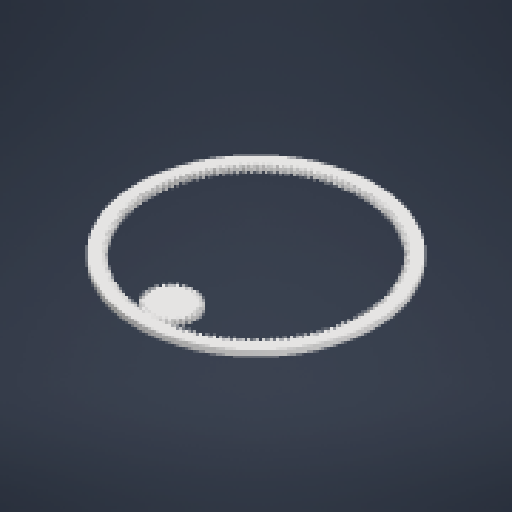
# Autodesk Inventor part: gears1
Saved by Autodesk Inventor 2026.1 (Build 301233000, 233)
## iProperties
Created: 2026-03-26
Part Number: gears1
Material: Generic
Document SubType Name: Modeling
Designer: sniel
Density: 1 g/cm^3
Appearance: Default
Author: sniel
Autodesk Inventor part; units mm, degrees
(part 1 of 2)
ref_plane "YZ Plane" through (0, 0, 0) normal (1, 0, 0) x (0, 1, 0)
ref_plane "XZ Plane" through (0, 0, 0) normal (0, 1, 0) x (-1, 0, 0)
ref_plane "XY Plane" through (0, 0, 0) normal (0, 0, 1) x (1, 0, 0)
sketch "Sketch2" plane through (0, 0, 0) normal (0, 1, 0) x (-1, 0, 0)
  arc A0 (4.4637, 88.5451) -> (4.2983, 91.7831) centre (-8.532, 89.5045) ccw
  arc A1 (4.2983, 91.7831) -> (3.1779, 92.0382) centre (-0.6449, 72.6571) ccw
  arc A2 (3.1779, 92.0382) -> (1.6272, 89.1908) centre (13.7576, 84.4303) ccw
  arc A3 (1.6272, 89.1908) -> (0.662, 89.295) centre (-0.6449, 72.6571) ccw
  arc A4 (0.662, 89.295) -> (-0.2457, 92.4075) centre (-12.2047, 87.2315) ccw
  arc A5 (-0.2457, 92.4075) -> (-1.3947, 92.3973) centre (-0.6449, 72.6571) ccw
  arc A6 (-1.3947, 92.3973) -> (-2.247, 89.2692) centre (10.6543, 87.4344) ccw
  arc A7 (-2.247, 89.2692) -> (-3.2102, 89.1479) centre (-0.6449, 72.6571) ccw
  arc A8 (-3.2102, 89.1479) -> (-4.8112, 91.9672) centre (-15.2542, 84.1728) ccw
  arc A9 (-4.8112, 91.9672) -> (-5.9269, 91.6923) centre (-0.6449, 72.6571) ccw
  arc A10 (-5.9269, 91.6923) -> (-6.0348, 88.4519) centre (6.9418, 89.6419) ccw
  arc A11 (-6.0348, 88.4519) -> (-6.9441, 88.1118) centre (-0.6449, 72.6571) ccw
  arc A12 (-6.9441, 88.1118) -> (-9.1521, 90.4859) centre (-17.5161, 80.4933) ccw
  arc A13 (-9.1521, 90.4859) -> (-10.1744, 89.9611) centre (-0.6449, 72.6571) ccw
  arc A14 (-10.1744, 89.9611) -> (-9.532, 86.7832) centre (2.8204, 90.9337) ccw
  arc A15 (-9.532, 86.7832) -> (-10.3384, 86.2425) centre (-0.6449, 72.6571) ccw
  arc A16 (-10.3384, 86.2425) -> (-13.0344, 88.0435) centre (-18.8684, 76.3913) ccw
  arc A17 (-13.0344, 88.0435) -> (-13.9081, 87.2971) centre (-0.6449, 72.6571) ccw
  arc A18 (-13.9081, 87.2971) -> (-12.5502, 84.3529) centre (-1.4879, 91.2402) ccw
  arc A19 (-12.5502, 84.3529) -> (-13.2101, 83.6409) centre (-0.6449, 72.6571) ccw
  arc A20 (-13.2101, 83.6409) -> (-16.2488, 84.7715) centre (-19.2384, 72.088) ccw
  arc A21 (-16.2488, 84.7715) -> (-16.9267, 83.8437) centre (-0.6449, 72.6571) ccw
  arc A22 (-16.9267, 83.8437) -> (-14.9265, 81.2921) centre (-5.7507, 90.5449) ccw
  arc A23 (-14.9265, 81.2921) -> (-15.4044, 80.4471) centre (-0.6449, 72.6571) ccw
  arc A24 (-15.4044, 80.4471) -> (-18.6219, 80.8465) centre (-18.6059, 67.8154) ccw
  arc A25 (-18.6219, 80.8465) -> (-19.0677, 79.7874) centre (-0.6449, 72.6571) ccw
  arc A26 (-19.0677, 79.7874) -> (-16.5329, 77.7658) centre (-9.7383, 88.8852) ccw
  arc A27 (-16.5329, 77.7658) -> (-16.8031, 76.8333) centre (-0.6449, 72.6571) ccw
  arc A28 (-16.8031, 76.8333) -> (-20.0259, 76.48) centre (-17.0052, 63.8038) ccw
  arc A29 (-20.0259, 76.48) -> (-20.2154, 75.3466) centre (-0.6449, 72.6571) ccw
  arc A30 (-20.2154, 75.3466) -> (-17.2828, 73.9641) centre (-13.2356, 86.3507) ccw
  arc A31 (-17.2828, 73.9641) -> (-17.3306, 72.9944) centre (-0.6449, 72.6571) ccw
  arc A32 (-17.3306, 72.9944) -> (-20.3851, 71.9073) centre (-14.5225, 60.2695) ccw
  arc A33 (-20.3851, 71.9073) -> (-20.3081, 70.7608) centre (-0.6449, 72.6571) ccw
  arc A34 (-20.3081, 70.7608) -> (-17.1357, 70.0919) centre (-16.0542, 83.078) ccw
  arc A35 (-17.1357, 70.0919) -> (-16.9586, 69.1374) centre (-0.6449, 72.6571) ccw
  arc A36 (-16.9586, 69.1374) -> (-19.6801, 67.3751) centre (-11.2917, 57.403) ccw
  arc A37 (-19.6801, 67.3751) -> (-19.3408, 66.2773) centre (-0.6449, 72.6571) ccw
  arc A38 (-19.3408, 66.2773) -> (-16.0996, 66.358) centre (-18.0421, 79.2435) ccw
  arc A39 (-16.0996, 66.358) -> (-15.7072, 65.47) centre (-0.6449, 72.6571) ccw
  arc A40 (-15.7072, 65.47) -> (-17.9489, 63.1277) centre (-7.4868, 55.3589) ccw
  arc A41 (-17.9489, 63.1277) -> (-17.3655, 62.1377) centre (-0.6449, 72.6571) ccw
  arc A42 (-17.3655, 62.1377) -> (-14.2303, 62.9637) centre (-19.092, 75.0539) ccw
  arc A43 (-14.2303, 62.9637) -> (-13.6437, 62.1902) centre (-0.6449, 72.6571) ccw
  arc A44 (-13.6437, 62.1902) -> (-15.2848, 59.394) centre (-3.3132, 54.2473) ccw
  arc A45 (-15.2848, 59.394) -> (-14.4889, 58.5652) centre (-0.6449, 72.6571) ccw
  arc A46 (-14.4889, 58.5652) -> (-11.6287, 60.092) centre (-19.1475, 70.7351) ccw
  arc A47 (-11.6287, 60.092) -> (-10.8795, 59.4746) centre (-0.6449, 72.6571) ccw
  arc A48 (-10.8795, 59.4746) -> (-11.8315, 56.3753) centre (1.0043, 54.1282) ccw
  arc A49 (-11.8315, 56.3753) -> (-10.8659, 55.7524) centre (-0.6449, 72.6571) ccw
  arc A50 (-10.8659, 55.7524) -> (-8.4349, 57.8976) centre (-18.2055, 66.5199) ccw
  arc A51 (-8.4349, 57.8976) -> (-7.5635, 57.4697) centre (-0.6449, 72.6571) ccw
  arc A52 (-7.5635, 57.4697) -> (-7.7751, 54.2344) centre (5.233, 55.008) ccw
  arc A53 (-7.7751, 54.2344) -> (-6.6919, 53.851) centre (-0.6449, 72.6571) ccw
  arc A54 (-6.6919, 53.851) -> (-4.8211, 56.499) centre (-16.3168, 62.6356) ccw
  arc A55 (-4.8211, 56.499) -> (-3.8746, 56.2835) centre (-0.6449, 72.6571) ccw
  arc A56 (-3.8746, 56.2835) -> (-3.3344, 53.0866) centre (9.1447, 56.8393) ccw
  arc A57 (-3.3344, 53.0866) -> (-2.1919, 52.9634) centre (-0.6449, 72.6571) ccw
  arc A58 (-2.1919, 52.9634) -> (-0.9822, 55.9715) centre (-13.5833, 59.2915) ccw
  arc A59 (-0.9822, 55.9715) -> (-0.0115, 55.9801) centre (-0.6449, 72.6571) ccw
  arc A60 (-0.0115, 55.9801) -> (1.2514, 52.9939) centre (12.5286, 59.5233) ccw
  arc A61 (1.2514, 52.9939) -> (2.3915, 53.1375) centre (-0.6449, 72.6571) ccw
  arc A62 (2.3915, 53.1375) -> (2.8748, 56.3434) centre (-10.1522, 56.668) ccw
  arc A63 (2.8748, 56.3434) -> (3.8174, 56.5757) centre (-0.6449, 72.6571) ccw
  arc A64 (3.8174, 56.5757) -> (5.7349, 53.9613) centre (15.2024, 62.9154) ccw
  arc A65 (5.7349, 53.9613) -> (6.8112, 54.3639) centre (-0.6449, 72.6571) ccw
  arc A66 (6.8112, 54.3639) -> (6.5422, 57.5949) centre (-6.2086, 54.9065) ccw
  arc A67 (6.5422, 57.5949) -> (7.4058, 58.0383) centre (-0.6449, 72.6571) ccw
  arc A68 (7.4058, 58.0383) -> (9.8745, 55.9365) centre (17.0219, 66.8326) ccw
  arc A69 (9.8745, 55.9365) -> (10.8289, 56.5765) centre (-0.6449, 72.6571) ccw
  arc A70 (10.8289, 56.5765) -> (9.822, 59.6583) centre (-1.965, 54.1019) ccw
  arc A71 (9.822, 59.6583) -> (10.5601, 60.2889) centre (-0.6449, 72.6571) ccw
  arc A72 (10.5601, 60.2889) -> (13.447, 58.8132) centre (17.8889, 71.0638) ccw
  arc A73 (13.447, 58.8132) -> (14.2281, 59.656) centre (-0.6449, 72.6571) ccw
  arc A74 (14.2281, 59.656) -> (12.5376, 62.4226) centre (2.3497, 54.2976) ccw
  arc A75 (12.5376, 62.4226) -> (13.1104, 63.2064) centre (-0.6449, 72.6571) ccw
  arc A76 (13.1104, 63.2064) -> (16.2598, 62.4362) centre (17.7567, 75.381) ccw
  arc A77 (16.2598, 62.4362) -> (16.8255, 63.4364) centre (-0.6449, 72.6571) ccw
  arc A78 (16.8255, 63.4364) -> (14.5425, 65.7386) centre (6.503, 55.4831) ccw
  arc A79 (14.5425, 65.7386) -> (14.9191, 66.6333) centre (-0.6449, 72.6571) ccw
  arc A80 (14.9191, 66.6333) -> (18.1612, 66.6102) centre (16.6326, 79.5513) ccw
  arc A81 (18.1612, 66.6102) -> (18.481, 67.7139) centre (-0.6449, 72.6571) ccw
  arc A82 (18.481, 67.7139) -> (15.7287, 69.4275) centre (10.2709, 57.5944) ccw
  arc A83 (15.7287, 69.4275) -> (15.8888, 70.385) centre (-0.6449, 72.6571) ccw
  arc A84 (15.8888, 70.385) -> (19.0488, 71.1102) centre (14.5769, 83.3499) ccw
  arc A85 (19.0488, 71.1102) -> (19.1055, 72.2579) centre (-0.6449, 72.6571) ccw
  arc A86 (19.1055, 72.2579) -> (16.0321, 73.2906) centre (13.4504, 60.5178) ccw
  arc A87 (16.0321, 73.2906) -> (15.9671, 74.2592) centre (-0.6449, 72.6571) ccw
  arc A88 (15.9671, 74.2592) -> (18.8748, 75.6936) centre (11.7007, 86.5721) ccw
  arc A89 (18.8748, 75.6936) -> (18.6652, 76.8234) centre (-0.6449, 72.6571) ccw
  arc A90 (18.6652, 76.8234) -> (15.4365, 77.1195) centre (15.8699, 64.0956) ccw
  arc A91 (15.4365, 77.1195) -> (15.1499, 78.047) centre (-0.6449, 72.6571) ccw
  arc A92 (15.1499, 78.047) -> (17.6484, 80.1133) centre (8.1589, 89.0441) ccw
  arc A93 (17.6484, 80.1133) -> (17.1839, 81.1643) centre (-0.6449, 72.6571) ccw
  arc A94 (17.1839, 81.1643) -> (13.974, 80.7079) centre (17.3992, 68.135) ccw
  arc A95 (13.974, 80.7079) -> (13.4811, 81.5443) centre (-0.6449, 72.6571) ccw
  arc A96 (13.4811, 81.5443) -> (15.4358, 84.131) centre (4.1425, 90.6327) ccw
  arc A97 (15.4358, 84.131) -> (14.7414, 85.0466) centre (-0.6449, 72.6571) ccw
  arc A98 (14.7414, 85.0466) -> (11.7233, 83.8622) centre (17.9557, 72.4182) ccw
  arc A99 (11.7233, 83.8622) -> (11.0508, 84.5624) centre (-0.6449, 72.6571) ccw
  arc A100 (11.0508, 84.5624) -> (12.3562, 87.5302) centre (-0.132, 91.2522) ccw
  arc A101 (12.3562, 87.5302) -> (11.4695, 88.261) centre (-0.6449, 72.6571) ccw
  arc A102 (11.4695, 88.261) -> (8.8058, 86.4125) centre (17.5094, 76.7142) ccw
  arc A103 (8.8058, 86.4125) -> (7.99, 86.9387) centre (-0.6449, 72.6571) ccw
  arc A104 (7.99, 86.9387) -> (8.5758, 90.1276) centre (-4.4341, 90.8693) ccw
  arc A105 (8.5758, 90.1276) -> (7.5444, 90.6341) centre (-0.6449, 72.6571) ccw
  arc A106 (7.5444, 90.6341) -> (5.3789, 88.2212) centre (16.0845, 80.7915) ccw
  arc A107 (5.3789, 88.2212) -> (4.4637, 88.5451) centre (-0.6449, 72.6571) ccw
  arc A108 (5.0279, 89.5592) -> (4.1055, 92.6747) centre (-14.5226, 85.4651) ccw
  arc A109 (6.0853, 89.4936) -> (5.0279, 89.5592) centre (0, 0) ccw
  arc A110 (7.3858, 92.4711) -> (6.0853, 89.4936) centre (24.9795, 83.0134) ccw
  arc A111 (8.4774, 92.3774) -> (7.3858, 92.4711) centre (0, 0) ccw
  arc A112 (9.2517, 89.2219) -> (8.4774, 92.3774) centre (-10.4704, 86.0556) ccw
  arc A113 (10.3048, 89.1064) -> (9.2517, 89.2219) centre (0, 0) ccw
  arc A114 (11.7445, 92.0191) -> (10.3048, 89.1064) centre (28.8719, 81.7411) ccw
  arc A115 (12.8304, 91.874) -> (11.7445, 92.0191) centre (0, 0) ccw
  arc A116 (13.4548, 88.6854) -> (12.8304, 91.874) centre (-6.3948, 86.4541) ccw
  arc A117 (14.5013, 88.5203) -> (13.4548, 88.6854) centre (0, 0) ccw
  arc A118 (16.0769, 91.3618) -> (14.5013, 88.5203) centre (32.6998, 80.2865) ccw
  arc A119 (17.1548, 91.1656) -> (16.0769, 91.3618) centre (0, 0) ccw
  arc A120 (17.6279, 87.9511) -> (17.1548, 91.1656) centre (-2.3049, 86.6596) ccw
  arc A121 (18.6654, 87.7367) -> (17.6279, 87.9511) centre (0, 0) ccw
  arc A122 (20.3735, 90.5007) -> (18.6654, 87.7367) centre (36.4548, 78.6527) ccw
  arc A123 (21.4409, 90.2538) -> (20.3735, 90.5007) centre (0, 0) ccw
  arc A124 (21.7617, 87.0205) -> (21.4409, 90.2538) centre (1.7901, 86.6718) ccw
  arc A125 (22.7879, 86.7574) -> (21.7617, 87.0205) centre (0, 0) ccw
  arc A126 (24.6246, 89.4376) -> (22.7879, 86.7574) centre (40.1285, 76.8434) ccw
  arc A127 (25.6792, 89.1405) -> (24.6246, 89.4376) centre (0, 0) ccw
  arc A128 (25.8469, 85.8957) -> (25.6792, 89.1405) centre (5.8812, 86.4905) ccw
  arc A129 (26.8595, 85.5844) -> (25.8469, 85.8957) centre (0, 0) ccw
  arc A130 (28.8208, 88.1749) -> (26.8595, 85.5844) centre (43.7126, 74.8626) ccw
  arc A131 (29.8601, 87.8284) -> (28.8208, 88.1749) centre (0, 0) ccw
  arc A132 (29.8744, 84.5793) -> (29.8601, 87.8284) centre (9.9591, 86.1163) ccw
  arc A133 (30.8712, 84.2205) -> (29.8744, 84.5793) centre (0, 0) ccw
  arc A134 (32.9526, 86.7155) -> (30.8712, 84.2205) centre (47.1992, 72.7148) ccw
  arc A135 (33.9745, 86.3203) -> (32.9526, 86.7155) centre (0, 0) ccw
  arc A136 (33.8353, 83.0741) -> (33.9745, 86.3203) centre (14.0147, 85.5499) ccw
  arc A137 (34.8141, 82.6687) -> (33.8353, 83.0741) centre (0, 0) ccw
  arc A138 (37.011, 85.0626) -> (34.8141, 82.6687) centre (50.5804, 70.4047) ccw
  arc A139 (38.013, 84.6195) -> (37.011, 85.0626) centre (0, 0) ccw
  arc A140 (37.7207, 81.3836) -> (38.013, 84.6195) centre (18.0392, 84.7926) ccw
  arc A141 (38.6792, 80.9324) -> (37.7207, 81.3836) centre (0, 0) ccw
  arc A142 (40.9867, 83.2198) -> (38.6792, 80.9324) centre (53.8488, 67.9375) ccw
  arc A143 (41.9667, 82.73) -> (40.9867, 83.2198) centre (0, 0) ccw
  arc A144 (41.5219, 79.5114) -> (41.9667, 82.73) centre (22.0233, 83.8461) ccw
  arc A145 (42.458, 79.0155) -> (41.5219, 79.5114) centre (0, 0) ccw
  arc A146 (44.871, 81.1914) -> (42.458, 79.0155) centre (56.9971, 65.3187) ccw
  arc A147 (45.8267, 80.6558) -> (44.871, 81.1914) centre (0, 0) ccw
  arc A148 (45.2304, 77.4619) -> (45.8267, 80.6558) centre (25.9583, 82.7125) ccw
  arc A149 (46.1421, 76.9223) -> (45.2304, 77.4619) centre (0, 0) ccw
  arc A150 (48.6551, 78.9818) -> (46.1421, 76.9223) centre (60.0181, 62.5542) ccw
  arc A151 (49.5845, 78.4017) -> (48.6551, 78.9818) centre (0, 0) ccw
  arc A152 (48.8381, 75.2395) -> (49.5845, 78.4017) centre (29.8354, 81.3944) ccw
  arc A153 (49.7233, 74.6574) -> (48.8381, 75.2395) centre (0, 0) ccw
  arc A154 (52.3307, 76.596) -> (49.7233, 74.6574) centre (62.9052, 59.6501) ccw
  arc A155 (53.2317, 75.9726) -> (52.3307, 76.596) centre (0, 0) ccw
  arc A156 (52.3367, 72.8492) -> (53.2317, 75.9726) centre (33.6459, 79.8946) ccw
  arc A157 (53.1934, 72.226) -> (52.3367, 72.8492) centre (0, 0) ccw
  arc A158 (55.8895, 74.0393) -> (53.1934, 72.226) centre (65.652, 56.6129) ccw
  arc A159 (56.7601, 73.374) -> (55.8895, 74.0393) centre (0, 0) ccw
  arc A160 (55.7186, 70.2963) -> (56.7601, 73.374) centre (37.3814, 78.2166) ccw
  arc A161 (56.5449, 69.6334) -> (55.7186, 70.2963) centre (0, 0) ccw
  arc A162 (59.3237, 71.3173) -> (56.5449, 69.6334) centre (68.2522, 53.4493) ccw
  arc A163 (60.1618, 70.6117) -> (59.3237, 71.3173) centre (0, 0) ccw
  arc A164 (58.9761, 67.5866) -> (60.1618, 70.6117) centre (41.0334, 76.364) ccw
  arc A165 (59.7702, 66.8854) -> (58.9761, 67.5866) centre (0, 0) ccw
  arc A166 (62.6254, 68.4362) -> (59.7702, 66.8854) centre (70.7002, 50.1665) ccw
  arc A167 (63.4293, 67.6918) -> (62.6254, 68.4362) centre (0, 0) ccw
  arc A168 (62.1021, 64.7261) -> (63.4293, 67.6918) centre (44.5939, 74.341) ccw
  arc A169 (62.8622, 63.9881) -> (62.1021, 64.7261) centre (0, 0) ccw
  arc A170 (65.7874, 65.4024) -> (62.8622, 63.9881) centre (72.9904, 46.7718) ccw
  arc A171 (66.5552, 64.6209) -> (65.7874, 65.4024) centre (0, 0) ccw
  arc A172 (65.0894, 61.7211) -> (66.5552, 64.6209) centre (48.0548, 72.1522) ccw
  arc A173 (65.8138, 60.9481) -> (65.0894, 61.7211) centre (0, 0) ccw
  arc A174 (68.8026, 62.2227) -> (65.8138, 60.9481) centre (75.1177, 43.2727) ccw
  arc A175 (69.5326, 61.4058) -> (68.8026, 62.2227) centre (0, 0) ccw
  arc A176 (67.9316, 58.5785) -> (69.5326, 61.4058) centre (51.4085, 69.8023) ccw
  arc A177 (68.6186, 57.7721) -> (67.9316, 58.5785) centre (0, 0) ccw
  arc A178 (71.6642, 58.9041) -> (68.6186, 57.7721) centre (77.0775, 39.677) ccw
  arc A179 (72.3549, 58.0536) -> (71.6642, 58.9041) centre (0, 0) ccw
  arc A180 (70.6221, 55.3051) -> (72.3549, 58.0536) centre (54.6476, 67.2967) ccw
  arc A181 (71.2703, 54.4672) -> (70.6221, 55.3051) centre (0, 0) ccw
  arc A182 (74.366, 55.4541) -> (71.2703, 54.4672) centre (78.8652, 35.9928) ccw
  arc A183 (75.0157, 54.5719) -> (74.366, 55.4541) centre (0, 0) ccw
  arc A184 (73.1551, 51.9083) -> (75.0157, 54.5719) centre (57.7646, 64.6409) ccw
  arc A185 (73.763, 51.0407) -> (73.1551, 51.9083) centre (0, 0) ccw
  arc A186 (76.9018, 51.8803) -> (73.763, 51.0407) centre (80.4769, 32.2283) ccw
  arc A187 (77.5092, 50.9685) -> (76.9018, 51.8803) centre (0, 0) ccw
  arc A188 (75.5248, 48.3957) -> (77.5092, 50.9685) centre (60.7528, 61.8409) ccw
  arc A189 (76.0911, 47.5003) -> (75.5248, 48.3957) centre (0, 0) ccw
  arc A190 (79.266, 48.1908) -> (76.0911, 47.5003) centre (81.9091, 28.3918) ccw
  arc A191 (79.8296, 47.2513) -> (79.266, 48.1908) centre (0, 0) ccw
  arc A192 (77.726, 44.7751) -> (79.8296, 47.2513) centre (63.6054, 58.9029) ccw
  arc A193 (78.2494, 43.854) -> (77.726, 44.7751) centre (0, 0) ccw
  arc A194 (81.4534, 44.3937) -> (78.2494, 43.854) centre (83.1585, 24.492) ccw
  arc A195 (81.972, 43.4286) -> (81.4534, 44.3937) centre (0, 0) ccw
  arc A196 (79.7537, 41.0545) -> (81.972, 43.4286) centre (66.3161, 55.8334) ccw
  arc A197 (80.233, 40.1098) -> (79.7537, 41.0545) centre (0, 0) ccw
  arc A198 (83.459, 40.4976) -> (80.233, 40.1098) centre (84.2224, 20.5376) ccw
  arc A199 (83.9314, 39.5091) -> (83.459, 40.4976) centre (0, 0) ccw
  arc A200 (81.6035, 37.2424) -> (83.9314, 39.5091) centre (68.8788, 52.6394) ccw
  arc A201 (82.0377, 36.2761) -> (81.6035, 37.2424) centre (0, 0) ccw
  arc A202 (85.2783, 36.5111) -> (82.0377, 36.2761) centre (85.0983, 16.5373) ccw
  arc A203 (85.7036, 35.5014) -> (85.2783, 36.5111) centre (0, 0) ccw
  arc A204 (83.2712, 33.3472) -> (85.7036, 35.5014) centre (71.2879, 49.3279) ccw
  arc A205 (83.6593, 32.3614) -> (83.2712, 33.3472) centre (0, 0) ccw
  arc A206 (86.9074, 32.4432) -> (83.6593, 32.3614) centre (85.7843, 12.5002) ccw
  arc A207 (87.2845, 31.4145) -> (86.9074, 32.4432) centre (0, 0) ccw
  arc A208 (84.7531, 29.3775) -> (87.2845, 31.4145) centre (73.5378, 45.9063) ccw
  arc A209 (85.0942, 28.3745) -> (84.7531, 29.3775) centre (0, 0) ccw
  arc A210 (88.3425, 28.3028) -> (85.0942, 28.3745) centre (86.2789, 8.4351) ccw
  arc A211 (88.6706, 27.2575) -> (88.3425, 28.3028) centre (0, 0) ccw
  arc A212 (86.0459, 25.3423) -> (88.6706, 27.2575) centre (75.6237, 42.3823) ccw
  arc A213 (86.3392, 24.3244) -> (86.0459, 25.3423) centre (0, 0) ccw
  arc A214 (89.5806, 24.0993) -> (86.3392, 24.3244) centre (86.581, 4.3512) ccw
  arc A215 (89.8589, 23.0397) -> (89.5806, 24.0993) centre (0, 0) ccw
  arc A216 (87.1467, 21.2506) -> (89.8589, 23.0397) centre (77.5408, 38.7638) ccw
  arc A217 (87.3916, 20.2199) -> (87.1467, 21.2506) centre (0, 0) ccw
  arc A218 (90.6187, 19.842) -> (87.3916, 20.2199) centre (86.6899, 0.2576) ccw
  arc A219 (90.8467, 18.7704) -> (90.6187, 19.842) centre (0, 0) ccw
  arc A220 (88.053, 17.1114) -> (90.8467, 18.7704) centre (79.2848, 35.0587) ccw
  arc A221 (88.249, 16.0703) -> (88.053, 17.1114) centre (0, 0) ccw
  arc A222 (91.4546, 15.5405) -> (88.249, 16.0703) centre (86.6053, -3.8365) ccw
  arc A223 (91.6318, 14.4593) -> (91.4546, 15.5405) centre (0, 0) ccw
  arc A224 (88.7628, 12.9341) -> (91.6318, 14.4593) centre (80.852, 31.2754) ccw
  arc A225 (88.9094, 11.8849) -> (88.7628, 12.9341) centre (0, 0) ccw
  arc A226 (92.0865, 11.2042) -> (88.9094, 11.8849) centre (86.3275, -7.9221) ccw
  arc A227 (92.2124, 10.1159) -> (92.0865, 11.2042) centre (0, 0) ccw
  arc A228 (89.2746, 8.7279) -> (92.2124, 10.1159) centre (82.2388, 27.4223) ccw
  arc A229 (89.3715, 7.6729) -> (89.2746, 8.7279) centre (0, 0) ccw
  arc A230 (92.5128, 6.843) -> (89.3715, 7.6729) centre (85.8571, -11.9901) ccw
  arc A231 (92.5872, 5.7499) -> (92.5128, 6.843) centre (0, 0) ccw
  arc A232 (89.5872, 4.5022) -> (92.5872, 5.7499) centre (83.442, 23.508) ccw
  arc A233 (89.6341, 3.4438) -> (89.5872, 4.5022) centre (0, 0) ccw
  arc A234 (92.7328, 2.4665) -> (89.6341, 3.4438) centre (85.1951, -16.0312) ccw
  arc A235 (92.7554, 1.3711) -> (92.7328, 2.4665) centre (0, 0) ccw
  arc A236 (89.6998, 0.2665) -> (92.7554, 1.3711) centre (84.4591, 19.5413) ccw
  arc A237 (89.6967, -0.7929) -> (89.6998, 0.2665) centre (0, 0) ccw
  arc A238 (92.7458, -1.9155) -> (89.6967, -0.7929) centre (84.3429, -20.0366) ccw
  arc A239 (92.7167, -3.0107) -> (92.7458, -1.9155) centre (0, 0) ccw
  arc A240 (89.6123, -3.9698) -> (92.7167, -3.0107) centre (85.2877, 15.531) ccw
  arc A241 (89.5592, -5.0279) -> (89.6123, -3.9698) centre (0, 0) ccw
  arc A242 (92.5519, -6.2932) -> (89.5592, -5.0279) centre (83.3026, -23.9973) ccw
  arc A243 (92.4711, -7.3858) -> (92.5519, -6.2932) centre (0, 0) ccw
  arc A244 (89.3249, -8.1973) -> (92.4711, -7.3858) centre (85.926, 11.486) ccw
  arc A245 (89.2219, -9.2517) -> (89.3249, -8.1973) centre (0, 0) ccw
  arc A246 (92.1514, -10.6569) -> (89.2219, -9.2517) centre (82.0764, -27.9045) ccw
  arc A247 (92.0191, -11.7445) -> (92.1514, -10.6569) centre (0, 0) ccw
  arc A248 (88.8381, -12.4065) -> (92.0191, -11.7445) centre (86.3725, 7.4154) ccw
  arc A249 (88.6854, -13.4548) -> (88.8381, -12.4065) centre (0, 0) ccw
  arc A250 (91.5453, -14.9968) -> (88.6854, -13.4548) centre (80.6671, -31.7494) ccw
  arc A251 (91.3618, -16.0769) -> (91.5453, -14.9968) centre (0, 0) ccw
  arc A252 (88.1531, -16.588) -> (91.3618, -16.0769) centre (86.6263, 3.3282) ccw
  arc A253 (87.9511, -17.6279) -> (88.1531, -16.588) centre (0, 0) ccw
  arc A254 (90.735, -19.3033) -> (87.9511, -17.6279) centre (79.0777, -35.5234) ccw
  arc A255 (90.5007, -20.3735) -> (90.735, -19.3033) centre (0, 0) ccw
  arc A256 (87.2714, -20.7324) -> (90.5007, -20.3735) centre (86.6869, -0.7664) ccw
  arc A257 (87.0205, -21.7617) -> (87.2714, -20.7324) centre (0, 0) ccw
  arc A258 (89.7222, -23.5666) -> (87.0205, -21.7617) centre (77.3119, -39.2182) ccw
  arc A259 (89.4376, -24.6246) -> (89.7222, -23.5666) centre (0, 0) ccw
  arc A260 (86.195, -24.8306) -> (89.4376, -24.6246) centre (86.5539, -4.8593) ccw
  arc A261 (85.8957, -25.8469) -> (86.195, -24.8306) centre (0, 0) ccw
  arc A262 (88.5091, -27.7774) -> (85.8957, -25.8469) centre (75.3736, -42.8254) ccw
  arc A263 (88.1749, -28.8208) -> (88.5091, -27.7774) centre (0, 0) ccw
  arc A264 (84.9262, -28.8734) -> (88.1749, -28.8208) centre (86.2279, -8.9413) ccw
  arc A265 (84.5793, -29.8744) -> (84.9262, -28.8734) centre (0, 0) ccw
  arc A266 (87.0986, -31.9262) -> (84.5793, -29.8744) centre (73.2671, -46.3371) ccw
  arc A267 (86.7155, -32.9526) -> (87.0986, -31.9262) centre (0, 0) ccw
  arc A268 (83.4679, -32.8518) -> (86.7155, -32.9526) centre (85.7094, -13.0034) ccw
  arc A269 (83.0741, -33.8353) -> (83.4679, -32.8518) centre (0, 0) ccw
  arc A270 (85.4937, -36.0038) -> (83.0741, -33.8353) centre (70.9971, -49.7454) ccw
  arc A271 (85.0626, -37.011) -> (85.4937, -36.0038) centre (0, 0) ccw
  arc A272 (81.8234, -36.7569) -> (85.0626, -37.011) centre (84.9997, -17.0365) ccw
  arc A273 (81.3836, -37.7207) -> (81.8234, -36.7569) centre (0, 0) ccw
  arc A274 (83.6981, -40.001) -> (81.3836, -37.7207) centre (68.5687, -53.0427) ccw
  arc A275 (83.2198, -40.9867) -> (83.6981, -40.001) centre (0, 0) ccw
  arc A276 (79.9963, -40.5799) -> (83.2198, -40.9867) centre (84.1004, -21.0315) ccw
  arc A277 (79.5114, -41.5219) -> (79.9963, -40.5799) centre (0, 0) ccw
  arc A278 (81.7157, -43.909) -> (79.5114, -41.5219) centre (65.9873, -56.2216) ccw
  arc A279 (81.1914, -44.871) -> (81.7157, -43.909) centre (0, 0) ccw
  arc A280 (77.9906, -44.3124) -> (81.1914, -44.871) centre (83.0133, -24.9797) ccw
  arc A281 (77.4619, -45.2304) -> (77.9906, -44.3124) centre (0, 0) ccw
  arc A282 (79.551, -47.719) -> (77.4619, -45.2304) centre (63.2586, -59.2751) ccw
  arc A283 (78.9818, -48.6551) -> (79.551, -47.719) centre (0, 0) ccw
  arc A284 (75.811, -47.9461) -> (78.9818, -48.6551) centre (81.7411, -28.872) ccw
  arc A285 (75.2395, -48.8381) -> (75.811, -47.9461) centre (0, 0) ccw
  arc A286 (77.2087, -51.4225) -> (75.2395, -48.8381) centre (60.3888, -62.1964) ccw
  arc A287 (76.596, -52.3307) -> (77.2087, -51.4225) centre (0, 0) ccw
  arc A288 (73.4622, -51.4727) -> (76.596, -52.3307) centre (80.2864, -32.7) ccw
  arc A289 (72.8492, -52.3367) -> (73.4622, -51.4727) centre (0, 0) ccw
  arc A290 (74.6942, -55.0112) -> (72.8492, -52.3367) centre (57.3843, -64.9788) ccw
  arc A291 (74.0393, -55.8895) -> (74.6942, -55.0112) centre (0, 0) ccw
  arc A292 (70.9495, -54.8845) -> (74.0393, -55.8895) centre (78.6526, -36.455) ccw
  arc A293 (70.2963, -55.7186) -> (70.9495, -54.8845) centre (0, 0) ccw
  arc A294 (72.013, -58.4772) -> (70.2963, -55.7186) centre (54.2517, -67.6162) ccw
  arc A295 (71.3173, -59.3237) -> (72.013, -58.4772) centre (0, 0) ccw
  arc A296 (68.2784, -58.1738) -> (71.3173, -59.3237) centre (76.8433, -40.1287) ccw
  arc A297 (67.5866, -58.9761) -> (68.2784, -58.1738) centre (0, 0) ccw
  arc A298 (69.1711, -61.8128) -> (67.5866, -58.9761) centre (50.998, -70.1028) ccw
  arc A299 (68.4362, -62.6254) -> (69.1711, -61.8128) centre (0, 0) ccw
  arc A300 (65.455, -61.3333) -> (68.4362, -62.6254) centre (74.8625, -43.7128) ccw
  arc A301 (64.7261, -62.1021) -> (65.455, -61.3333) centre (0, 0) ccw
  arc A302 (66.1748, -65.0104) -> (64.7261, -62.1021) centre (47.6305, -72.4329) ccw
  arc A303 (65.4024, -65.7874) -> (66.1748, -65.0104) centre (0, 0) ccw
  arc A304 (62.4855, -64.356) -> (65.4024, -65.7874) centre (72.7147, -47.1993) ccw
  arc A305 (61.7211, -65.0894) -> (62.4855, -64.356) centre (0, 0) ccw
  arc A306 (63.0309, -68.0629) -> (61.7211, -65.0894) centre (44.1568, -74.6014) ccw
  arc A307 (62.2227, -68.8026) -> (63.0309, -68.0629) centre (0, 0) ccw
  arc A308 (59.3767, -67.235) -> (62.2227, -68.8026) centre (70.4046, -50.5806) ccw
  arc A309 (58.5785, -67.9316) -> (59.3767, -67.235) centre (0, 0) ccw
  arc A310 (59.7463, -70.9636) -> (58.5785, -67.9316) centre (40.5845, -76.6035) ccw
  arc A311 (58.9041, -71.6642) -> (59.7463, -70.9636) centre (0, 0) ccw
  arc A312 (56.1353, -69.964) -> (58.9041, -71.6642) centre (67.9374, -53.849) ccw
  arc A313 (55.3051, -70.6221) -> (56.1353, -69.964) centre (0, 0) ccw
  arc A314 (56.3285, -73.7059) -> (55.3051, -70.6221) centre (36.9217, -78.4346) ccw
  arc A315 (55.4541, -74.366) -> (56.3285, -73.7059) centre (0, 0) ccw
  arc A316 (52.7686, -72.5369) -> (55.4541, -74.366) centre (65.3186, -56.9972) ccw
  arc A317 (51.9083, -73.1551) -> (52.7686, -72.5369) centre (0, 0) ccw
  arc A318 (52.7849, -76.2837) -> (51.9083, -73.1551) centre (33.1765, -80.0907) ccw
  arc A319 (51.8803, -76.9018) -> (52.7849, -76.2837) centre (0, 0) ccw
  arc A320 (49.2843, -74.9479) -> (51.8803, -76.9018) centre (62.5541, -60.0182) ccw
  arc A321 (48.3957, -75.5248) -> (49.2843, -74.9479) centre (0, 0) ccw
  arc A322 (49.1236, -78.6914) -> (48.3957, -75.5248) centre (29.3572, -81.5681) ccw
  arc A323 (48.1908, -79.266) -> (49.1236, -78.6914) centre (0, 0) ccw
  arc A324 (45.6899, -77.1918) -> (48.1908, -79.266) centre (59.6499, -62.9053) ccw
  arc A325 (44.7751, -77.726) -> (45.6899, -77.1918) centre (0, 0) ccw
  arc A326 (45.3526, -80.9234) -> (44.7751, -77.726) centre (25.4724, -82.8635) ccw
  arc A327 (44.3937, -81.4534) -> (45.3526, -80.9234) centre (0, 0) ccw
  arc A328 (41.9936, -79.2633) -> (44.3937, -81.4534) centre (56.6127, -65.6521) ccw
  arc A329 (41.0545, -79.7537) -> (41.9936, -79.2633) centre (0, 0) ccw
  arc A330 (41.4804, -82.9749) -> (41.0545, -79.7537) centre (21.5308, -83.9739) ccw
  arc A331 (40.4976, -83.459) -> (41.4804, -82.9749) centre (0, 0) ccw
  arc A332 (38.2036, -81.158) -> (40.4976, -83.459) centre (53.4492, -68.2524) ccw
  arc A333 (37.2424, -81.6035) -> (38.2036, -81.158) centre (0, 0) ccw
  arc A334 (37.5157, -84.8412) -> (37.2424, -81.6035) centre (17.5412, -84.897) ccw
  arc A335 (36.5111, -85.2783) -> (37.5157, -84.8412) centre (0, 0) ccw
  arc A336 (34.3283, -82.8716) -> (36.5111, -85.2783) centre (50.1664, -70.7003) ccw
  arc A337 (33.3472, -83.2712) -> (34.3283, -82.8716) centre (0, 0) ccw
  arc A338 (33.4673, -86.5182) -> (33.3472, -83.2712) centre (13.5124, -85.6307) ccw
  arc A339 (32.4432, -86.9074) -> (33.4673, -86.5182) centre (0, 0) ccw
  arc A340 (30.3764, -84.4003) -> (32.4432, -86.9074) centre (46.7716, -72.9905) ccw
  arc A341 (29.3775, -84.7531) -> (30.3764, -84.4003) centre (0, 0) ccw
  arc A342 (29.3442, -88.0021) -> (29.3775, -84.7531) centre (9.4535, -86.1733) ccw
  arc A343 (28.3028, -88.3425) -> (29.3442, -88.0021) centre (0, 0) ccw
  arc A344 (26.3568, -85.7406) -> (28.3028, -88.3425) centre (43.2725, -75.1178) ccw
  arc A345 (25.3423, -86.0459) -> (26.3568, -85.7406) centre (0, 0) ccw
  arc A346 (25.1556, -89.2897) -> (25.3423, -86.0459) centre (5.3735, -86.5235) ccw
  arc A347 (24.0993, -89.5806) -> (25.1556, -89.2897) centre (0, 0) ccw
  arc A348 (22.2783, -86.8896) -> (24.0993, -89.5806) centre (39.6768, -77.0775) ccw
  arc A349 (21.2506, -87.1467) -> (22.2783, -86.8896) centre (0, 0) ccw
  arc A350 (20.9109, -90.378) -> (21.2506, -87.1467) centre (1.2814, -86.6808) ccw
  arc A351 (19.842, -90.6187) -> (20.9109, -90.378) centre (0, 0) ccw
  arc A352 (18.1502, -87.8448) -> (19.842, -90.6187) centre (35.9926, -78.8653) ccw
  arc A353 (17.1114, -88.053) -> (18.1502, -87.8448) centre (0, 0) ccw
  arc A354 (16.6195, -91.2647) -> (17.1114, -88.053) centre (-2.8134, -86.6446) ccw
  arc A355 (15.5405, -91.4546) -> (16.6195, -91.2647) centre (0, 0) ccw
  arc A356 (13.9815, -88.6039) -> (15.5405, -91.4546) centre (32.2281, -80.477) ccw
  arc A357 (12.9341, -88.7628) -> (13.9815, -88.6039) centre (0, 0) ccw
  arc A358 (12.291, -91.9477) -> (12.9341, -88.7628) centre (-6.902, -86.415) ccw
  arc A359 (11.2042, -92.0865) -> (12.291, -91.9477) centre (0, 0) ccw
  arc A360 (9.7816, -89.1653) -> (11.2042, -92.0865) centre (28.3917, -81.9092) ccw
  arc A361 (8.7279, -89.2746) -> (9.7816, -89.1653) centre (0, 0) ccw
  arc A362 (7.9351, -92.4256) -> (8.7279, -89.2746) centre (-10.9752, -85.9927) ccw
  arc A363 (6.843, -92.5128) -> (7.9351, -92.4256) centre (0, 0) ccw
  arc A364 (5.5599, -89.5278) -> (6.843, -92.5128) centre (24.4919, -83.1586) ccw
  arc A365 (4.5022, -89.5872) -> (5.5599, -89.5278) centre (0, 0) ccw
  arc A366 (3.5615, -92.6972) -> (4.5022, -89.5872) centre (-15.024, -85.3784) ccw
  arc A367 (2.4665, -92.7328) -> (3.5615, -92.6972) centre (0, 0) ccw
  arc A368 (1.3258, -89.6904) -> (2.4665, -92.7328) centre (20.5374, -84.2224) ccw
  arc A369 (0.2665, -89.6998) -> (1.3258, -89.6904) centre (0, 0) ccw
  arc A370 (-0.82, -92.762) -> (0.2665, -89.6998) centre (-19.0391, -84.5737) ccw
  arc A371 (-1.9155, -92.7458) -> (-0.82, -92.762) centre (0, 0) ccw
  arc A372 (-2.9112, -89.653) -> (-1.9155, -92.7458) centre (16.5372, -85.0983) ccw
  arc A373 (-3.9698, -89.6123) -> (-2.9112, -89.653) centre (0, 0) ccw
  arc A374 (-5.1997, -92.6197) -> (-3.9698, -89.6123) centre (-23.0118, -83.5802) ccw
  arc A375 (-6.2932, -92.5519) -> (-5.1997, -92.6197) centre (0, 0) ccw
  arc A376 (-7.1418, -89.4155) -> (-6.2932, -92.5519) centre (12.5, -85.7843) ccw
  arc A377 (-8.1973, -89.3249) -> (-7.1418, -89.4155) centre (0, 0) ccw
  arc A378 (-9.5678, -92.2708) -> (-8.1973, -89.3249) centre (-26.9332, -82.4003) ccw
  arc A379 (-10.6569, -92.1514) -> (-9.5678, -92.2708) centre (0, 0) ccw
  arc A380 (-11.3564, -88.9785) -> (-10.6569, -92.1514) centre (8.4349, -86.2789) ccw
  arc A381 (-12.4065, -88.8381) -> (-11.3564, -88.9785) centre (0, 0) ccw
  arc A382 (-13.9146, -91.7161) -> (-12.4065, -88.8381) centre (-30.7944, -81.0364) ccw
  arc A383 (-14.9968, -91.5453) -> (-13.9146, -91.7161) centre (0, 0) ccw
  arc A384 (-15.5457, -88.3429) -> (-14.9968, -91.5453) centre (4.351, -86.581) ccw
  arc A385 (-16.588, -88.1531) -> (-15.5457, -88.3429) centre (0, 0) ccw
  arc A386 (-18.2303, -90.9566) -> (-16.588, -88.1531) centre (-34.587, -79.4917) ccw
  arc A387 (-19.3033, -90.735) -> (-18.2303, -90.9566) centre (0, 0) ccw
  arc A388 (-19.7003, -87.5102) -> (-19.3033, -90.735) centre (0.2575, -86.6899) ccw
  arc A389 (-20.7324, -87.2714) -> (-19.7003, -87.5102) centre (0, 0) ccw
  arc A390 (-22.5053, -89.9942) -> (-20.7324, -87.2714) centre (-38.3024, -77.7697) ccw
  arc A391 (-23.5666, -89.7222) -> (-22.5053, -89.9942) centre (0, 0) ccw
  arc A392 (-23.8109, -86.4822) -> (-23.5666, -89.7222) centre (-3.8367, -86.6053) ccw
  arc A393 (-24.8306, -86.195) -> (-23.8109, -86.4822) centre (0, 0) ccw
  arc A394 (-26.7302, -88.831) -> (-24.8306, -86.195) centre (-41.9322, -75.8741) ccw
  arc A395 (-27.7774, -88.5091) -> (-26.7302, -88.831) centre (0, 0) ccw
  arc A396 (-27.8684, -85.2613) -> (-27.7774, -88.5091) centre (-7.9223, -86.3275) ccw
  arc A397 (-28.8734, -84.9262) -> (-27.8684, -85.2613) centre (0, 0) ccw
  arc A398 (-30.8953, -87.4696) -> (-28.8734, -84.9262) centre (-45.4686, -73.8093) ccw
  arc A399 (-31.9262, -87.0986) -> (-30.8953, -87.4696) centre (0, 0) ccw
  arc A400 (-31.8638, -83.8501) -> (-31.9262, -87.0986) centre (-11.9902, -85.857) ccw
  arc A401 (-32.8518, -83.4679) -> (-31.8638, -83.8501) centre (0, 0) ccw
  arc A402 (-34.9916, -85.913) -> (-32.8518, -83.4679) centre (-48.9034, -71.5797) ccw
  arc A403 (-36.0038, -85.4937) -> (-34.9916, -85.913) centre (0, 0) ccw
  arc A404 (-35.788, -82.2518) -> (-36.0038, -85.4937) centre (-16.0314, -85.195) ccw
  arc A405 (-36.7569, -81.8234) -> (-35.788, -82.2518) centre (0, 0) ccw
  arc A406 (-39.0097, -84.1647) -> (-36.7569, -81.8234) centre (-52.2292, -69.1904) ccw
  arc A407 (-40.001, -83.6981) -> (-39.0097, -84.1647) centre (0, 0) ccw
  arc A408 (-39.6323, -80.4699) -> (-40.001, -83.6981) centre (-20.0368, -84.3429) ccw
  arc A409 (-40.5799, -79.9963) -> (-39.6323, -80.4699) centre (0, 0) ccw
  arc A410 (-42.9408, -82.2286) -> (-40.5799, -79.9963) centre (-55.4384, -66.6467) ccw
  arc A411 (-43.909, -81.7157) -> (-42.9408, -82.2286) centre (0, 0) ccw
  arc A412 (-43.3883, -78.5085) -> (-43.909, -81.7157) centre (-23.9975, -83.3026) ccw
  arc A413 (-44.3124, -77.9906) -> (-43.3883, -78.5085) centre (0, 0) ccw
  arc A414 (-46.7761, -80.109) -> (-44.3124, -77.9906) centre (-58.5239, -63.9543) ccw
  arc A415 (-47.719, -79.551) -> (-46.7761, -80.109) centre (0, 0) ccw
  arc A416 (-47.0474, -76.372) -> (-47.719, -79.551) centre (-27.9047, -82.0764) ccw
  arc A417 (-47.9461, -75.811) -> (-47.0474, -76.372) centre (0, 0) ccw
  arc A418 (-50.507, -77.8106) -> (-47.9461, -75.811) centre (-61.4788, -61.1192) ccw
  arc A419 (-51.4225, -77.2087) -> (-50.507, -77.8106) centre (0, 0) ccw
  arc A420 (-50.6015, -74.065) -> (-51.4225, -77.2087) centre (-31.7495, -80.667) ccw
  arc A421 (-51.4727, -73.4622) -> (-50.6015, -74.065) centre (0, 0) ccw
  arc A422 (-54.1252, -75.3386) -> (-51.4727, -73.4622) centre (-64.2965, -58.1477) ccw
  arc A423 (-55.0112, -74.6942) -> (-54.1252, -75.3386) centre (0, 0) ccw
  arc A424 (-54.0427, -71.5927) -> (-55.0112, -74.6942) centre (-35.5236, -79.0777) ccw
  arc A425 (-54.8845, -70.9495) -> (-54.0427, -71.5927) centre (0, 0) ccw
  arc A426 (-57.6227, -72.6986) -> (-54.8845, -70.9495) centre (-66.9708, -55.0464) ccw
  arc A427 (-58.4772, -72.013) -> (-57.6227, -72.6986) centre (0, 0) ccw
  arc A428 (-57.3634, -68.9607) -> (-58.4772, -72.013) centre (-39.2183, -77.3118) ccw
  arc A429 (-58.1738, -68.2784) -> (-57.3634, -68.9607) centre (0, 0) ccw
  arc A430 (-60.9915, -69.8963) -> (-58.1738, -68.2784) centre (-69.4956, -51.8224) ccw
  arc A431 (-61.8128, -69.1711) -> (-60.9915, -69.8963) centre (0, 0) ccw
  arc A432 (-60.556, -66.1748) -> (-61.8128, -69.1711) centre (-42.8256, -75.3735) ccw
  arc A433 (-61.3333, -65.455) -> (-60.556, -66.1748) centre (0, 0) ccw
  arc A434 (-64.2243, -66.938) -> (-61.3333, -65.455) centre (-71.8654, -48.4827) ccw
  arc A435 (-65.0104, -66.1748) -> (-64.2243, -66.938) centre (0, 0) ccw
  arc A436 (-63.6135, -63.2412) -> (-65.0104, -66.1748) centre (-46.3373, -73.267) ccw
  arc A437 (-64.356, -62.4855) -> (-63.6135, -63.2412) centre (0, 0) ccw
  arc A438 (-67.3137, -63.8303) -> (-64.356, -62.4855) centre (-74.0747, -45.0348) ccw
  arc A439 (-68.0629, -63.0309) -> (-67.3137, -63.8303) centre (0, 0) ccw
  arc A440 (-66.5291, -60.1666) -> (-68.0629, -63.0309) centre (-49.7456, -70.997) ccw
  arc A441 (-67.235, -59.3767) -> (-66.5291, -60.1666) centre (0, 0) ccw
  arc A442 (-70.253, -60.5803) -> (-67.235, -59.3767) centre (-76.1188, -41.4864) ccw
  arc A443 (-70.9636, -59.7463) -> (-70.253, -60.5803) centre (0, 0) ccw
  arc A444 (-69.2962, -56.9577) -> (-70.9636, -59.7463) centre (-53.0428, -68.5686) ccw
  arc A445 (-69.964, -56.1353) -> (-69.2962, -56.9577) centre (0, 0) ccw
  arc A446 (-73.0355, -57.195) -> (-69.964, -56.1353) centre (-77.9931, -37.8454) ccw
  arc A447 (-73.7059, -56.3285) -> (-73.0355, -57.195) centre (0, 0) ccw
  arc A448 (-71.9086, -53.6216) -> (-73.7059, -56.3285) centre (-56.2218, -65.9872) ccw
  arc A449 (-72.5369, -52.7686) -> (-71.9086, -53.6216) centre (0, 0) ccw
  arc A450 (-75.655, -53.6822) -> (-72.5369, -52.7686) centre (-79.6933, -34.12) ccw
  arc A451 (-76.2837, -52.7849) -> (-75.655, -53.6822) centre (0, 0) ccw
  arc A452 (-74.3607, -50.166) -> (-76.2837, -52.7849) centre (-59.2753, -63.2585) ccw
  arc A453 (-74.9479, -49.2843) -> (-74.3607, -50.166) centre (0, 0) ccw
  arc A454 (-78.1057, -50.0495) -> (-74.9479, -49.2843) centre (-81.2157, -30.3185) ccw
  arc A455 (-78.6914, -49.1236) -> (-78.1057, -50.0495) centre (0, 0) ccw
  arc A456 (-76.6468, -46.5984) -> (-78.6914, -49.1236) centre (-62.1965, -60.3887) ccw
  arc A457 (-77.1918, -45.6899) -> (-76.6468, -46.5984) centre (0, 0) ccw
  arc A458 (-80.3821, -46.3052) -> (-77.1918, -45.6899) centre (-82.5568, -26.4493) ccw
  arc A459 (-80.9234, -45.3526) -> (-80.3821, -46.3052) centre (0, 0) ccw
  arc A460 (-78.7618, -42.9268) -> (-80.9234, -45.3526) centre (-64.9789, -57.3841) ccw
  arc A461 (-79.2633, -41.9936) -> (-78.7618, -42.9268) centre (0, 0) ccw
  arc A462 (-82.4792, -42.4575) -> (-79.2633, -41.9936) centre (-83.7138, -22.5211) ccw
  arc A463 (-82.9749, -41.4804) -> (-82.4792, -42.4575) centre (0, 0) ccw
  arc A464 (-80.7011, -39.1594) -> (-82.9749, -41.4804) centre (-67.6163, -54.2515) ccw
  arc A465 (-81.158, -38.2036) -> (-80.7011, -39.1594) centre (0, 0) ccw
  arc A466 (-84.3922, -38.5151) -> (-81.158, -38.2036) centre (-84.6839, -18.5426) ccw
  arc A467 (-84.8412, -37.5157) -> (-84.3922, -38.5151) centre (0, 0) ccw
  arc A468 (-82.4604, -35.3046) -> (-84.8412, -37.5157) centre (-70.1029, -50.9979) ccw
  arc A469 (-82.8716, -34.3283) -> (-82.4604, -35.3046) centre (0, 0) ccw
  arc A470 (-86.1169, -34.4868) -> (-82.8716, -34.3283) centre (-85.4651, -14.5228) ccw
  arc A471 (-86.5182, -33.4673) -> (-86.1169, -34.4868) centre (0, 0) ccw
  arc A472 (-84.0356, -31.3711) -> (-86.5182, -33.4673) centre (-72.433, -47.6304) ccw
  arc A473 (-84.4003, -30.3764) -> (-84.0356, -31.3711) centre (0, 0) ccw
  arc A474 (-87.6494, -30.3815) -> (-84.4003, -30.3764) centre (-86.0556, -10.4706) ccw
  arc A475 (-88.0021, -29.3442) -> (-87.6494, -30.3815) centre (0, 0) ccw
  arc A476 (-85.4233, -27.3676) -> (-88.0021, -29.3442) centre (-74.6015, -44.1566) ccw
  arc A477 (-85.7406, -26.3568) -> (-85.4233, -27.3676) centre (0, 0) ccw
  arc A478 (-88.9864, -26.2084) -> (-85.7406, -26.3568) centre (-86.4541, -6.3949) ccw
  arc A479 (-89.2897, -25.1556) -> (-88.9864, -26.2084) centre (0, 0) ccw
  arc A480 (-86.6205, -23.303) -> (-89.2897, -25.1556) centre (-76.6036, -40.5844) ccw
  arc A481 (-86.8896, -22.2783) -> (-86.6205, -23.303) centre (0, 0) ccw
  arc A482 (-90.1248, -21.9768) -> (-86.8896, -22.2783) centre (-86.6596, -2.3051) ccw
  arc A483 (-90.378, -20.9109) -> (-90.1248, -21.9768) centre (0, 0) ccw
  arc A484 (-87.6243, -19.1864) -> (-90.378, -20.9109) centre (-78.4347, -36.9215) ccw
  arc A485 (-87.8448, -18.1502) -> (-87.6243, -19.1864) centre (0, 0) ccw
  arc A486 (-91.0621, -17.6962) -> (-87.8448, -18.1502) centre (-86.6718, 1.79) ccw
  arc A487 (-91.2647, -16.6195) -> (-91.0621, -17.6962) centre (0, 0) ccw
  arc A488 (-88.4326, -15.027) -> (-91.2647, -16.6195) centre (-80.0908, -33.1763) ccw
  arc A489 (-88.6039, -13.9815) -> (-88.4326, -15.027) centre (0, 0) ccw
  arc A490 (-91.7962, -13.3761) -> (-88.6039, -13.9815) centre (-86.4905, 5.881) ccw
  arc A491 (-91.9477, -12.291) -> (-91.7962, -13.3761) centre (0, 0) ccw
  arc A492 (-89.0436, -10.834) -> (-91.9477, -12.291) centre (-81.5681, -29.357) ccw
  arc A493 (-89.1653, -9.7816) -> (-89.0436, -10.834) centre (0, 0) ccw
  arc A494 (-92.3254, -9.0261) -> (-89.1653, -9.7816) centre (-86.1163, 9.9589) ccw
  arc A495 (-92.4256, -7.9351) -> (-92.3254, -9.0261) centre (0, 0) ccw
  arc A496 (-89.4559, -6.6169) -> (-92.4256, -7.9351) centre (-82.8635, -25.4723) ccw
  arc A497 (-89.5278, -5.5599) -> (-89.4559, -6.6169) centre (0, 0) ccw
  arc A498 (-92.6487, -4.6561) -> (-89.5278, -5.5599) centre (-85.5499, 14.0146) ccw
  arc A499 (-92.6972, -3.5615) -> (-92.6487, -4.6561) centre (0, 0) ccw
  arc A500 (-89.6685, -2.385) -> (-92.6972, -3.5615) centre (-83.974, -21.5307) ccw
  arc A501 (-89.6904, -1.3258) -> (-89.6685, -2.385) centre (0, 0) ccw
  arc A502 (-92.7652, -0.2756) -> (-89.6904, -1.3258) centre (-84.7926, 18.039) ccw
  arc A503 (-92.762, 0.82) -> (-92.7652, -0.2756) centre (0, 0) ccw
  arc A504 (-89.6811, 1.8522) -> (-92.762, 0.82) centre (-84.8971, -17.541) ccw
  arc A505 (-89.653, 2.9112) -> (-89.6811, 1.8522) centre (0, 0) ccw
  arc A506 (-92.6747, 4.1055) -> (-89.653, 2.9112) centre (-83.8462, 22.0231) ccw
  arc A507 (-92.6197, 5.1997) -> (-92.6747, 4.1055) centre (0, 0) ccw
  arc A508 (-89.4936, 6.0853) -> (-92.6197, 5.1997) centre (-85.6307, -13.5122) ccw
  arc A509 (-89.4155, 7.1418) -> (-89.4936, 6.0853) centre (0, 0) ccw
  arc A510 (-92.3774, 8.4774) -> (-89.4155, 7.1418) centre (-82.7126, 25.9582) ccw
  arc A511 (-92.2708, 9.5678) -> (-92.3774, 8.4774) centre (0, 0) ccw
  arc A512 (-89.1064, 10.3048) -> (-92.2708, 9.5678) centre (-86.1733, -9.4533) ccw
  arc A513 (-88.9785, 11.3564) -> (-89.1064, 10.3048) centre (0, 0) ccw
  arc A514 (-91.874, 12.8304) -> (-88.9785, 11.3564) centre (-81.3944, 29.8352) ccw
  arc A515 (-91.7161, 13.9146) -> (-91.874, 12.8304) centre (0, 0) ccw
  arc A516 (-88.5203, 14.5013) -> (-91.7161, 13.9146) centre (-86.5236, -5.3733) ccw
  arc A517 (-88.3429, 15.5457) -> (-88.5203, 14.5013) centre (0, 0) ccw
  arc A518 (-91.1656, 17.1548) -> (-88.3429, 15.5457) centre (-79.8947, 33.6458) ccw
  arc A519 (-90.9566, 18.2303) -> (-91.1656, 17.1548) centre (0, 0) ccw
  arc A520 (-87.7367, 18.6654) -> (-90.9566, 18.2303) centre (-86.6808, -1.2813) ccw
  arc A521 (-87.5102, 19.7003) -> (-87.7367, 18.6654) centre (0, 0) ccw
  arc A522 (-90.2538, 21.4409) -> (-87.5102, 19.7003) centre (-78.2166, 37.3812) ccw
  arc A523 (-89.9942, 22.5053) -> (-90.2538, 21.4409) centre (0, 0) ccw
  arc A524 (-86.7574, 22.7879) -> (-89.9942, 22.5053) centre (-86.6446, 2.8136) ccw
  arc A525 (-86.4822, 23.8109) -> (-86.7574, 22.7879) centre (0, 0) ccw
  arc A526 (-89.1405, 25.6792) -> (-86.4822, 23.8109) centre (-76.3641, 41.0332) ccw
  arc A527 (-88.831, 26.7302) -> (-89.1405, 25.6792) centre (0, 0) ccw
  arc A528 (-85.5844, 26.8595) -> (-88.831, 26.7302) centre (-86.415, 6.9022) ccw
  arc A529 (-85.2613, 27.8684) -> (-85.5844, 26.8595) centre (0, 0) ccw
  arc A530 (-87.8284, 29.8601) -> (-85.2613, 27.8684) centre (-74.3411, 44.5937) ccw
  arc A531 (-87.4696, 30.8953) -> (-87.8284, 29.8601) centre (0, 0) ccw
  arc A532 (-84.2205, 30.8712) -> (-87.4696, 30.8953) centre (-85.9927, 10.9754) ccw
  arc A533 (-83.8501, 31.8638) -> (-84.2205, 30.8712) centre (0, 0) ccw
  arc A534 (-86.3203, 33.9745) -> (-83.8501, 31.8638) centre (-72.1523, 48.0547) ccw
  arc A535 (-85.913, 34.9916) -> (-86.3203, 33.9745) centre (0, 0) ccw
  arc A536 (-82.6687, 34.8141) -> (-85.913, 34.9916) centre (-85.3784, 15.0241) ccw
  arc A537 (-82.2518, 35.788) -> (-82.6687, 34.8141) centre (0, 0) ccw
  arc A538 (-84.6195, 38.013) -> (-82.2518, 35.788) centre (-69.8024, 51.4084) ccw
  arc A539 (-84.1647, 39.0097) -> (-84.6195, 38.013) centre (0, 0) ccw
  arc A540 (-80.9324, 38.6792) -> (-84.1647, 39.0097) centre (-84.5737, 19.0393) ccw
  arc A541 (-80.4699, 39.6323) -> (-80.9324, 38.6792) centre (0, 0) ccw
  arc A542 (-82.73, 41.9667) -> (-80.4699, 39.6323) centre (-67.2968, 54.6474) ccw
  arc A543 (-82.2286, 42.9408) -> (-82.73, 41.9667) centre (0, 0) ccw
  arc A544 (-79.0155, 42.458) -> (-82.2286, 42.9408) centre (-83.5802, 23.012) ccw
  arc A545 (-78.5085, 43.3883) -> (-79.0155, 42.458) centre (0, 0) ccw
  arc A546 (-80.6558, 45.8267) -> (-78.5085, 43.3883) centre (-64.641, 57.7645) ccw
  arc A547 (-80.109, 46.7761) -> (-80.6558, 45.8267) centre (0, 0) ccw
  arc A548 (-76.9223, 46.1421) -> (-80.109, 46.7761) centre (-82.4002, 26.9334) ccw
  arc A549 (-76.372, 47.0474) -> (-76.9223, 46.1421) centre (0, 0) ccw
  arc A550 (-78.4017, 49.5845) -> (-76.372, 47.0474) centre (-61.841, 60.7527) ccw
  arc A551 (-77.8106, 50.507) -> (-78.4017, 49.5845) centre (0, 0) ccw
  arc A552 (-74.6574, 49.7233) -> (-77.8106, 50.507) centre (-81.0363, 30.7946) ccw
  arc A553 (-74.065, 50.6015) -> (-74.6574, 49.7233) centre (0, 0) ccw
  arc A554 (-75.9726, 53.2317) -> (-74.065, 50.6015) centre (-58.903, 63.6053) ccw
  arc A555 (-75.3386, 54.1252) -> (-75.9726, 53.2317) centre (0, 0) ccw
  arc A556 (-72.226, 53.1934) -> (-75.3386, 54.1252) centre (-79.4917, 34.5872) ccw
  arc A557 (-71.5927, 54.0427) -> (-72.226, 53.1934) centre (0, 0) ccw
  arc A558 (-73.374, 56.7601) -> (-71.5927, 54.0427) centre (-55.8335, 66.316) ccw
  arc A559 (-72.6986, 57.6227) -> (-73.374, 56.7601) centre (0, 0) ccw
  arc A560 (-69.6334, 56.5449) -> (-72.6986, 57.6227) centre (-77.7696, 38.3025) ccw
  arc A561 (-68.9607, 57.3634) -> (-69.6334, 56.5449) centre (0, 0) ccw
  arc A562 (-70.6117, 60.1618) -> (-68.9607, 57.3634) centre (-52.6395, 68.8787) ccw
  arc A563 (-69.8963, 60.9915) -> (-70.6117, 60.1618) centre (0, 0) ccw
  arc A564 (-66.8854, 59.7702) -> (-69.8963, 60.9915) centre (-75.8741, 41.9324) ccw
  arc A565 (-66.1748, 60.556) -> (-66.8854, 59.7702) centre (0, 0) ccw
  arc A566 (-67.6918, 63.4293) -> (-66.1748, 60.556) centre (-49.328, 71.2878) ccw
  arc A567 (-66.938, 64.2243) -> (-67.6918, 63.4293) centre (0, 0) ccw
  arc A568 (-63.9881, 62.8622) -> (-66.938, 64.2243) centre (-73.8092, 45.4687) ccw
  arc A569 (-63.2412, 63.6135) -> (-63.9881, 62.8622) centre (0, 0) ccw
  arc A570 (-64.6209, 66.5552) -> (-63.2412, 63.6135) centre (-45.9065, 73.5377) ccw
  arc A571 (-63.8303, 67.3137) -> (-64.6209, 66.5552) centre (0, 0) ccw
  arc A572 (-60.9481, 65.8138) -> (-63.8303, 67.3137) centre (-71.5796, 48.9036) ccw
  arc A573 (-60.1666, 66.5291) -> (-60.9481, 65.8138) centre (0, 0) ccw
  arc A574 (-61.4058, 69.5326) -> (-60.1666, 66.5291) centre (-42.3825, 75.6236) ccw
  arc A575 (-60.5803, 70.253) -> (-61.4058, 69.5326) centre (0, 0) ccw
  arc A576 (-57.7721, 68.6186) -> (-60.5803, 70.253) centre (-69.1903, 52.2293) ccw
  arc A577 (-56.9577, 69.2962) -> (-57.7721, 68.6186) centre (0, 0) ccw
  arc A578 (-58.0536, 72.3549) -> (-56.9577, 69.2962) centre (-38.7639, 77.5407) ccw
  arc A579 (-57.195, 73.0355) -> (-58.0536, 72.3549) centre (0, 0) ccw
  arc A580 (-54.4672, 71.2703) -> (-57.195, 73.0355) centre (-66.6466, 55.4385) ccw
  arc A581 (-53.6216, 71.9086) -> (-54.4672, 71.2703) centre (0, 0) ccw
  arc A582 (-54.5719, 75.0157) -> (-53.6216, 71.9086) centre (-35.0588, 79.2848) ccw
  arc A583 (-53.6822, 75.655) -> (-54.5719, 75.0157) centre (0, 0) ccw
  arc A584 (-51.0407, 73.763) -> (-53.6822, 75.655) centre (-63.9542, 58.524) ccw
  arc A585 (-50.166, 74.3607) -> (-51.0407, 73.763) centre (0, 0) ccw
  arc A586 (-50.9685, 77.5092) -> (-50.166, 74.3607) centre (-31.2756, 80.8519) ccw
  arc A587 (-50.0495, 78.1057) -> (-50.9685, 77.5092) centre (0, 0) ccw
  arc A588 (-47.5003, 76.0911) -> (-50.0495, 78.1057) centre (-61.1191, 61.4789) ccw
  arc A589 (-46.5984, 76.6468) -> (-47.5003, 76.0911) centre (0, 0) ccw
  arc A590 (-47.2513, 79.8296) -> (-46.5984, 76.6468) centre (-27.4225, 82.2387) ccw
  arc A591 (-46.3052, 80.3821) -> (-47.2513, 79.8296) centre (0, 0) ccw
  arc A592 (-43.854, 78.2494) -> (-46.3052, 80.3821) centre (-58.1476, 64.2967) ccw
  arc A593 (-42.9268, 78.7618) -> (-43.854, 78.2494) centre (0, 0) ccw
  arc A594 (-43.4286, 81.972) -> (-42.9268, 78.7618) centre (-23.5082, 83.442) ccw
  arc A595 (-42.4575, 82.4792) -> (-43.4286, 81.972) centre (0, 0) ccw
  arc A596 (-40.1098, 80.233) -> (-42.4575, 82.4792) centre (-55.0463, 66.9709) ccw
  arc A597 (-39.1594, 80.7011) -> (-40.1098, 80.233) centre (0, 0) ccw
  arc A598 (-39.5091, 83.9314) -> (-39.1594, 80.7011) centre (-19.5415, 84.459) ccw
  arc A599 (-38.5151, 84.3922) -> (-39.5091, 83.9314) centre (0, 0) ccw
  arc A600 (-36.2761, 82.0377) -> (-38.5151, 84.3922) centre (-51.8222, 69.4957) ccw
  arc A601 (-35.3046, 82.4604) -> (-36.2761, 82.0377) centre (0, 0) ccw
  arc A602 (-35.5014, 85.7036) -> (-35.3046, 82.4604) centre (-15.5311, 85.2876) ccw
  arc A603 (-34.4868, 86.1169) -> (-35.5014, 85.7036) centre (0, 0) ccw
  arc A604 (-32.3614, 83.6593) -> (-34.4868, 86.1169) centre (-48.4825, 71.8655) ccw
  arc A605 (-31.3711, 84.0356) -> (-32.3614, 83.6593) centre (0, 0) ccw
  arc A606 (-31.4145, 87.2845) -> (-31.3711, 84.0356) centre (-11.4862, 85.9259) ccw
  arc A607 (-30.3815, 87.6494) -> (-31.4145, 87.2845) centre (0, 0) ccw
  arc A608 (-28.3745, 85.0942) -> (-30.3815, 87.6494) centre (-45.0346, 74.0748) ccw
  arc A609 (-27.3676, 85.4233) -> (-28.3745, 85.0942) centre (0, 0) ccw
  arc A610 (-27.2575, 88.6706) -> (-27.3676, 85.4233) centre (-7.4155, 86.3725) ccw
  arc A611 (-26.2084, 88.9864) -> (-27.2575, 88.6706) centre (0, 0) ccw
  arc A612 (-24.3244, 86.3392) -> (-26.2084, 88.9864) centre (-41.4862, 76.1189) ccw
  arc A613 (-23.303, 86.6205) -> (-24.3244, 86.3392) centre (0, 0) ccw
  arc A614 (-23.0397, 89.8589) -> (-23.303, 86.6205) centre (-3.3284, 86.6263) ccw
  arc A615 (-21.9768, 90.1248) -> (-23.0397, 89.8589) centre (0, 0) ccw
  arc A616 (-20.2199, 87.3916) -> (-21.9768, 90.1248) centre (-37.8453, 77.9932) ccw
  arc A617 (-19.1864, 87.6243) -> (-20.2199, 87.3916) centre (0, 0) ccw
  arc A618 (-18.7704, 90.8467) -> (-19.1864, 87.6243) centre (0.7662, 86.6869) ccw
  arc A619 (-17.6962, 91.0621) -> (-18.7704, 90.8467) centre (0, 0) ccw
  arc A620 (-16.0703, 88.249) -> (-17.6962, 91.0621) centre (-34.1199, 79.6934) ccw
  arc A621 (-15.027, 88.4326) -> (-16.0703, 88.249) centre (0, 0) ccw
  arc A622 (-14.4593, 91.6318) -> (-15.027, 88.4326) centre (4.8591, 86.554) ccw
  arc A623 (-13.3761, 91.7962) -> (-14.4593, 91.6318) centre (0, 0) ccw
  arc A624 (-11.8849, 88.9094) -> (-13.3761, 91.7962) centre (-30.3183, 81.2157) ccw
  arc A625 (-10.834, 89.0436) -> (-11.8849, 88.9094) centre (0, 0) ccw
  arc A626 (-10.1159, 92.2124) -> (-10.834, 89.0436) centre (8.9411, 86.2279) ccw
  arc A627 (-9.0261, 92.3254) -> (-10.1159, 92.2124) centre (0, 0) ccw
  arc A628 (-7.6729, 89.3715) -> (-9.0261, 92.3254) centre (-26.4491, 82.5569) ccw
  arc A629 (-6.6169, 89.4559) -> (-7.6729, 89.3715) centre (0, 0) ccw
  arc A630 (-5.7499, 92.5872) -> (-6.6169, 89.4559) centre (13.0032, 85.7095) ccw